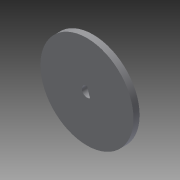
# Autodesk Inventor part: driveGearCap
Saved by Autodesk Inventor 2013 (Build 170138000, 138)
## iProperties
Created: 2014-07-02
Part Number: driveGearCap
Material: Generic
Document SubType Name: Modeling
Designer: Nano
Density: 1 g/cm^3
Author: Nano
Autodesk Inventor part; units mm, degrees
ref_plane "YZ Plane" through (0, 0, 0) normal (1, 0, 0) x (0, 1, 0)
ref_plane "XZ Plane" through (0, 0, 0) normal (0, 1, 0) x (-1, 0, 0)
ref_plane "XY Plane" through (0, 0, 0) normal (0, 0, 1) x (1, 0, 0)
sketch "Sketch1" plane through (0, 0, 0) normal (0, 0, 1) x (1, 0, 0)
  arc A0 (0, 2.5) -> (1.4504, -2.0363) centre (0, 0) ccw construction
  line L0 (0, 2.5) -> (1.4504, -2.0363) construction
  arc A1 (0.0854, 2.615) -> (1.5867, -2.0804) centre (0, 0) ccw
  line L1 (0.0854, 2.615) -> (1.5867, -2.0804)
  circle A2 centre (0, 0) radius 24.13
  dimension "d0" = 48.26
  constraints: 2 centre point, 2 end point, 2 point on circle, 1 other
  measures "d0" diameter of A2
extrude "Extrusion1" add sketch "Sketch1" along normal blind 3.175
body "Solid1"
